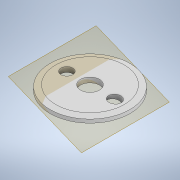
# Autodesk Inventor part: KF160
Saved by Autodesk Inventor 2021 (Build 250183000, 183)
## iProperties
Created: 2024-01-29
Part Number: KF160
Material: Generic
Document SubType Name: Modeling
Designer: Sebastián
Density: 1 g/cm^3
Appearance: Default
Author: Sebastián
Autodesk Inventor part; units mm, degrees
ref_plane "XZ Plane" through (0, 0, 0) normal (0, 1, 0) x (-1, 0, 0)
ref_plane "XY Plane" through (0, 0, 0) normal (0, 0, 1) x (1, 0, 0)
sketch "Sketch1" plane through (0, 0, 0) normal (1, 0, 0) x (0, 1, 0)
  line L0 (0, 95) -> (8.4, 95)
  line L1 (8.4, 95) -> (12, 81.5646)
  line L2 (12, 81.5646) -> (12, 0)
  line L3 (12, 0) -> (0, 0)
  line L4 (0, 0) -> (0, 73.5)
  line L5 (0, 73.5) -> (3.5, 73.5)
  line L6 (3.5, 73.5) -> (3.5, 76.5)
  line L7 (3.5, 76.5) -> (0, 76.5)
  line L8 (0, 76.5) -> (0, 95)
  line L9 (0, 114) -> (0, -19) construction
  line L10 (-2.4, 0) -> (14.4, 0) projected
  dimension "d0" = 95
  dimension "d1" = 12
  dimension "d2" = 8.4
  dimension "d3" = 3.5
  dimension "d4" = 3
  dimension "d5" = 73.5
  dimension "d6" = 165
  constraints: 19 end point, 6 perpendicular, 3 point on line, 1 horizontal
  measures "d0" distance of L3.end L0.start
  measures "d1" distance of L3.end L2.end
  measures "d2" distance of L0.start L0.end
  measures "d3" distance of L4.end L5.end
  measures "d4" distance of L5.end L6.end
  measures "d5" distance of L3.end L4.end
  measures "d6" angle of L2 L1
revolve "Revolution1" add sketch "Sketch1" angle 360 about axis through (0, -10, 0) along (0, 1, 0)
sketch "Sketch2" plane through (0, 12, 0) normal (0, 1, 0) x (1, 0, 0)
  circle A0 centre (0, 0) radius 22.5
  circle A1 centre (54.5, 0) radius 2.5
  dimension "d8" = 45
  dimension "d12" = 5
  dimension "d13" = 54.5
  constraints: 2 centre point, 1 coincident
  measures "d8" diameter of A0
  measures "d12" diameter of A1
  measures "d13" distance of A1.centre point (0, 0)
extrude "Extrusion1" cut sketch "Sketch2" against normal through all
ref_plane "Work Plane1" through (0, 0, 0) normal (0.3746, 0.9272, 0) x (0, 0, 1)
sketch "Sketch3" plane through (0, 0, 0) normal (0.3746, 0.9272, 0) x (0, 0, 1)
  ellipse E0 centre (0, 50.5315) end of major axis (-2.5, 50.5315) minor radius 2.318 projected
  circle A0 centre (0, 50.5315) radius 14
  point P0 (0, 0)
  dimension "d14" = 28
  constraints: 1 centre point, 1 coincident, 1 other
  measures "d14" diameter of A0
extrude "Extrusion2" cut sketch "Sketch3" along normal blind 73 contours E0 | A0
sketch "Sketch4" plane through (0, 0, 0) normal (0, -1, 0) x (1, 0, 0)
  line L0 (-48.75, -48.75) -> (-48.75, 48.75) construction
  line L1 (-48.75, 48.75) -> (48.75, 48.75) construction
  line L2 (48.75, 48.75) -> (48.75, -48.75) construction
  line L3 (48.75, -48.75) -> (-48.75, -48.75) construction
  line L4 (0, 133) -> (0, -133) construction
  circle A0 centre (48.75, 48.75) radius 5
  circle A1 centre (-48.75, 48.75) radius 5
  circle A2 centre (-48.75, -48.75) radius 5
  circle A3 centre (48.75, -48.75) radius 5
  point P0 (0, 0)
  point P1 (0, 0)
  dimension "d17" = 97.5
  dimension "d18" = 10
  constraints: 8 end point, 5 coincident, 4 centre point, 3 equal radius, 1 parallel, 9 other
  measures "d17" distance of L0.start L0.end
  measures "d18" diameter of A0
extrude "Extrusion3" cut sketch "Sketch4" against normal blind 0.5
sketch "Sketch5" plane through (0, 0, 0) normal (0, -1, 0) x (1, 0, 0)
  circle A0 centre (-55, 0) radius 14
  point P0 (0, 0)
  dimension "d21" = 28
  dimension "d22" = 55
  constraints: 1 centre point
  measures "d21" diameter of A0
  measures "d22" distance of point (0, 0) A0.centre
extrude "Extrusion4" cut sketch "Sketch5" against normal through all
body "Solid1"
